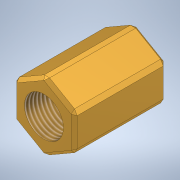
# Autodesk Inventor part: 5302_Brass_Nut_0.5_20_Tx_Rx_Relative_Positioning_MPSv2_v1
Saved by Autodesk Inventor 2021 (Build 250183000, 183)
## iProperties
Created: 2020-11-11
Part Number: 5302_Brass_Nut_0.5_20_Tx_Rx_Relative_Positioning_MPSv2_v1
Material: Brass, Soft Yellow
Document SubType Name: Modeling
Designer: Admin
Density: 8.47 g/cm^3
Appearance: Brass - Satin
Author: Admin
Autodesk Inventor part; units mm, degrees
ref_plane "YZ Plane" through (0, 0, 0) normal (1, 0, 0) x (0, 1, 0)
ref_plane "XZ Plane" through (0, 0, 0) normal (0, 1, 0) x (-1, 0, 0)
ref_plane "XY Plane" through (0, 0, 0) normal (0, 0, 1) x (1, 0, 0)
sketch "Sketch2" plane through (0, 0, 0) normal (0, 0, 1) x (1, 0, 0)
  circle A0 centre (0, 0) radius 6.35
  line L0 (0, 0) -> (0, 11.35)
  line L1 (0, 11.35) -> (9.8294, 5.675)
  line L2 (9.8294, 5.675) -> (9.8294, -5.675)
  line L3 (9.8294, -5.675) -> (0, -11.35)
  line L4 (0, -11.35) -> (-9.8294, -5.675)
  line L5 (-9.8294, -5.675) -> (-9.8294, 5.675)
  line L6 (-9.8294, 5.675) -> (0, 11.35)
  dimension "d11" = 12.7
  constraints: 14 end point, 4 parallel, 2 coincident, 1 centre point, 1 point on line, 1 vertical
  measures "d11" diameter of A0
extrude "Extrusion2" add sketch "Sketch2" along normal blind 30
thread "Thread2" size "1/2-20 UNF" class "2B" standard "ANSI Unified Screw Threads" full length
chamfer "Chamfer2" distance 1 angle 45 18 edges at (4.9147, 8.5125, 30) (9.8294, 0, 30) (4.9147, -8.5125, 30) (-4.9147, -8.5125, 30) (-9.8294, 0, 30) (-4.9147, 8.5125, 30) (9.8294, 5.675, 15) (9.8294, -5.675, 15) (0, -11.35, 15) (-9.8294, -5.675, 15) (-9.8294, 5.675, 15) (0, 11.35, 15) (-4.9147, 8.5125, 0) (4.9147, 8.5125, 0) (9.8294, 0, 0) (4.9147, -8.5125, 0) (-4.9147, -8.5125, 0) (-9.8294, 0, 0)
body "Solid2"
